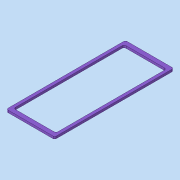
# Autodesk Inventor part: TopCoverContactSpacer
Saved by Autodesk Inventor 2018 (Build 220112000, 112)
## iProperties
Created: 2019-08-15
Part Number: TopCoverContactSpacer
Material: ABS Plastic
Document SubType Name: Modeling
Designer: Derek Wider
Density: 1.06 g/cm^3
Appearance: Violet
Author: Derek Wider
Autodesk Inventor part; units mm, degrees
ref_plane "YZ Plane" through (0, 0, 0) normal (1, 0, 0) x (0, 1, 0)
ref_plane "XZ Plane" through (0, 0, 0) normal (0, 1, 0) x (-1, 0, 0)
ref_plane "XY Plane" through (0, 0, 0) normal (0, 0, 1) x (1, 0, 0)
sketch "Sketch1" plane through (0, 0, 0) normal (0, 1, 0) x (-1, 0, 0)
  line L0 (0, 0) -> (38.1, 0)
  line L1 (38.1, 0) -> (38.1, -93.98)
  line L2 (38.1, -93.98) -> (0, -93.98)
  line L3 (0, -93.98) -> (0, 0)
  dimension "d0" = 38.1
  dimension "d1" = 93.98
  constraints: 8 end point, 2 parallel, 1 horizontal, 1 perpendicular
  measures "d0" distance of L1.end L2.end
  measures "d1" distance of L0.end L1.end
extrude "Extrusion1" add sketch "Sketch1" along normal blind 1.778
fillet "Fillet1" radius 1.27 4 edges at (0, 0.889, 0) (0, 0.889, -93.98) (-38.1, 0.889, -93.98) (-38.1, 0.889, 0)
sketch "Sketch3" plane through (0, 1.778, 0) normal (0, 1, 0) x (1, 0, 0)
  arc A0 (-38.1, 1.27) -> (-36.83, 0) centre (-36.83, 1.27) ccw projected
  line L0 (-36.83, 0) -> (-1.27, 0) projected
  arc A1 (-1.27, 0) -> (0, 1.27) centre (-1.27, 1.27) ccw projected
  line L1 (0, 1.27) -> (0, 92.71) projected
  arc A2 (0, 92.71) -> (-1.27, 93.98) centre (-1.27, 92.71) ccw projected
  line L2 (-1.27, 93.98) -> (-36.83, 93.98) projected
  arc A3 (-36.83, 93.98) -> (-38.1, 92.71) centre (-36.83, 92.71) ccw projected
  line L3 (-38.1, 92.71) -> (-38.1, 1.27) projected
  line L4 (-35.814, 2.286) -> (-2.286, 2.286)
  line L5 (-2.286, 4.826) -> (-2.286, 89.154)
  line L6 (-2.286, 91.694) -> (-35.814, 91.694)
  line L7 (-35.814, 89.154) -> (-35.814, 4.826)
  line L8 (-34.29, 3.302) -> (-3.81, 3.302)
  line L9 (-34.29, 90.678) -> (-3.81, 90.678)
  arc A4 (-35.814, 4.826) -> (-34.29, 3.302) centre (-34.29, 4.826) ccw
  arc A5 (-3.81, 3.302) -> (-2.286, 4.826) centre (-3.81, 4.826) ccw
  arc A6 (-2.286, 89.154) -> (-3.81, 90.678) centre (-3.81, 89.154) ccw
  arc A7 (-34.29, 90.678) -> (-35.814, 89.154) centre (-34.29, 89.154) ccw
  point P0 (0, 0)
  dimension "d9" = 2.286
  dimension "d10" = 1.016
  dimension "d11" = 1.016
  dimension "d12" = 1.524
  constraints: 12 end point, 8 point on circle, 8 tangent, 4 centre point, 4 point on line, 3 equal radius, 2 perpendicular, 3 other
  measures "d9" distance between parallel lines of L3 L7
  measures "d10" distance between parallel lines of L4 L8
  measures "d11" distance between parallel lines of L6 L9
  measures "d12" radius of A4
extrude "Extrusion3" cut sketch "Sketch3" against normal through all contours A5 L8 A4 L7 A7 L9 A6 L5
body "Solid1"
